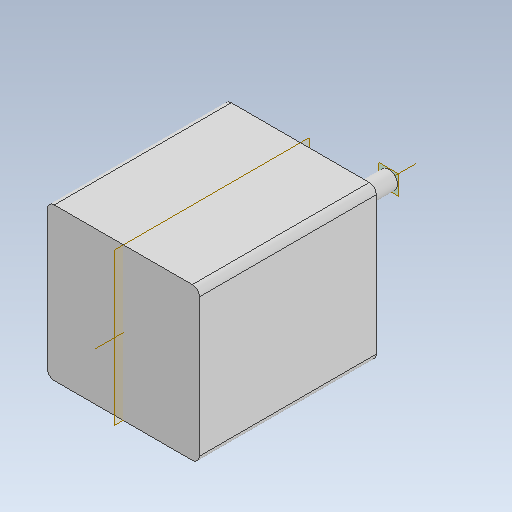
# Autodesk Inventor part: motor
Saved by Autodesk Inventor 2020 (Build 240168000, 168)
## iProperties
Created: 2022-12-14
Part Number: motor
Material: Generic
Document SubType Name: Modeling
Designer: Manish
Density: 1 g/cm^3
Appearance: Default
Author: Manish
Autodesk Inventor part; units mm, degrees
ref_plane "YZ Plane" through (0, 0, 0) normal (1, 0, 0) x (0, 1, 0)
ref_plane "XZ Plane" through (0, 0, 0) normal (0, 1, 0) x (-1, 0, 0)
ref_plane "XY Plane" through (0, 0, 0) normal (0, 0, 1) x (1, 0, 0)
sketch "Sketch1" plane through (0, 0, 0) normal (0, 0, 1) x (1, 0, 0)
  line L0 (0, -2) -> (0, -41)
  line L1 (2, -43) -> (41, -43)
  line L2 (43, -41) -> (43, -2)
  line L3 (41, 0) -> (2, 0)
  arc A0 (0, -41) -> (2, -43) centre (2, -41) ccw
  arc A1 (43, -2) -> (41, 0) centre (41, -2) ccw
  arc A2 (2, 0) -> (0, -2) centre (2, -2) ccw
  arc A3 (41, -43) -> (43, -41) centre (41, -41) ccw
  point P0 (0, 0)
  point P1 (0, -43)
  point P2 (43, -43)
  point P3 (43, 0)
  dimension "d0" = 43
  dimension "d1" = 43
  dimension "d7" = 2
  constraints: 8 end point, 8 point on circle, 8 point on line, 8 tangent, 4 centre point, 3 equal radius, 2 parallel, 1 perpendicular, 1 vertical
  measures "d0" distance of point (0, 0) point (0, -43)
  measures "d1" distance of point (43, -43) point (0, -43)
  measures "d7" radius of A0
extrude "Extrusion1" add sketch "Sketch1" along normal blind 50
sketch "Sketch2" plane through (0, 0, 0) normal (0, 0, -1) x (-1, 0, 0)
  line L0 (-43, -41) -> (-43, -2) projected
  line L1 (-2, -43) -> (-41, -43) projected
  line L2 (-43, 0) -> (0, -43)
  line L3 (0, -43) -> (0, 0)
  line L4 (0, 0) -> (-43, -43)
  circle A0 centre (-21.5, -21.5) radius 2.5
  circle A1 centre (-21.5, -21.5) radius 11
  dimension "d4" = 5
  dimension "d8" = 22
  constraints: 6 end point, 2 centre point, 2 perpendicular, 1 coincident, 1 midpoint
  measures "d4" diameter of A0
  measures "d8" diameter of A1
extrude "Extrusion2" add sketch "Sketch2" along normal blind 25 contours A0 L4 L2 | L2 L4 A0 | L4 A0 L2 | L2 A0 L4
ref_plane "Work Plane2" through (21.5, -41, 0) normal (1, 0, 0) x (0, 0, -1)
ref_plane "Work Plane3" through (21.5, -21.5, -25) normal (0, 0, -1) x (-1, 0, 0)
body "Solid1"
